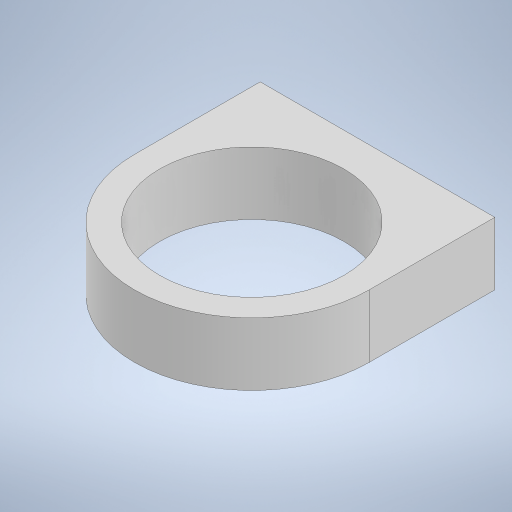
# Autodesk Inventor part: borde al borde
Saved by Autodesk Inventor 2024 (Build 280153000, 153)
## iProperties
Created: 2024-04-03
Part Number: borde al borde
Material: Generic
Document SubType Name: Modeling
Designer: compu
Density: 1 g/cm^3
Appearance: Default
Author: compu
Autodesk Inventor part; units mm, degrees
ref_plane "YZ Plane" through (0, 0, 0) normal (1, 0, 0) x (0, 1, 0)
ref_plane "XZ Plane" through (0, 0, 0) normal (0, 1, 0) x (-1, 0, 0)
ref_plane "XY Plane" through (0, 0, 0) normal (0, 0, 1) x (1, 0, 0)
sketch "Sketch1" plane through (0, 0, 0) normal (0, 1, 0) x (-1, 0, 0)
  circle A0 centre (0, 0) radius 4
  circle A1 centre (0, 0) radius 11
  circle A2 centre (0, 0) radius 14
  line L0 (14, 0) -> (14, -15)
  line L1 (14, -15) -> (-14, -15)
  line L2 (-14, -15) -> (-14, 0)
  line L3 (0, -20.8) -> (0, 19.8) projected
  dimension "d0" = 8
  dimension "d1" = 22
  dimension "d2" = 28
  dimension "d3" = 15
  constraints: 6 end point, 3 centre point, 3 coincident, 2 perpendicular, 2 point on circle, 1 tangent, 1 vertical
  measures "d0" diameter of A0
  measures "d1" diameter of A1
  measures "d2" diameter of A2
  measures "d3" distance from line of L1 point (0, 0)
extrude "Extrusion1" add sketch "Sketch1" along normal blind 7.5 contours L3 A2 A1 | A1 L3 A2 | L3 L1 L2 A2 | A2 L0 L1 L3
body "Solid1"
